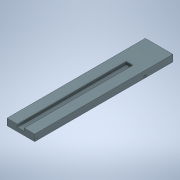
# Autodesk Inventor part: sina
Saved by Autodesk Inventor 2021.2 (Build 252289000, 289)
## iProperties
Created: 2024-04-19
Part Number: sina
Material: Lead
Document SubType Name: Modeling
Designer: cioba
Density: 11.34 g/cm^3
Appearance: Lead
Author: cioba
Autodesk Inventor part; units mm, degrees
ref_plane "YZ Plane" through (0, 0, 0) normal (1, 0, 0) x (0, 1, 0)
ref_plane "XZ Plane" through (0, 0, 0) normal (0, 1, 0) x (-1, 0, 0)
ref_plane "XY Plane" through (0, 0, 0) normal (0, 0, 1) x (1, 0, 0)
sketch "Sketch1" plane through (0, 0, 0) normal (0, 0, 1) x (1, 0, 0)
  line L0 (-7.378, 4.0507) -> (34.622, 4.0507)
  line L1 (34.622, 4.0507) -> (34.622, -5.9493)
  line L2 (34.622, -5.9493) -> (-7.378, -5.9493)
  line L3 (-7.378, -5.9493) -> (-7.378, 4.0507)
  line L4 (8.622, 4.0507) -> (8.622, 0.0507)
  line L5 (18.622, 4.0507) -> (18.622, 0.0507)
  line L6 (18.622, 0.0507) -> (8.622, 0.0507)
  point P0 (0, 0)
  constraints: 14 end point, 4 perpendicular, 2 parallel, 2 point on line, 1 horizontal
extrude "Extrusion1" add sketch "Sketch1" against normal blind 45
extrude "Extrusion2" add sketch "Sketch1" along normal blind 165 contours L0 L4 L6 L5 L1 L2 L3
sketch "Sketch2" plane through (34.622, -5.9493, -45) normal (1, 0, 0) x (0, 0, -1)
  line L0 (0, 0) -> (0, 10) projected
  line L1 (0, 0) -> (-210, 0) projected
  line L2 (-210, 10) -> (0, 10) projected
  circle A0 centre (-42.793, 2.5) radius 1.5
  point P0 (-45, 5.9493)
  constraints: 1 centre point
hole "Hole1" at (34.622, -3.4493, -2.207) direction (-1, 0, 0) diameter 3 depth 5 tip angle 118
sketch "Sketch3" plane through (34.622, -5.9493, -45) normal (1, 0, 0) x (0, 0, -1)
  line L0 (0, 0) -> (-210, 0) projected
  line L1 (-210, 0) -> (-207.5, 0)
  line L2 (-207.5, 0) -> (-207.5, 2.5)
  circle A0 centre (-207.5, 2.5) radius 1.5
  point P0 (-45, 5.9493)
  dimension "d19" = 2.5
  dimension "d20" = 2.5
  dimension "d21" = 3
  constraints: 4 end point, 1 centre point, 1 coincident, 1 perpendicular, 1 point on line
  measures "d19" distance of L0.end L1.end
  measures "d20" distance of L1.end L2.end
  measures "d21" diameter of A0
hole "Hole2" at (34.622, -3.4493, 162.5) direction (-1, 0, 0) diameter 3 depth 5 tip angle 118
sketch "Sketch4" plane through (-7.378, -5.9493, -45) normal (-1, 0, 0) x (0, 0, 1)
  circle A0 centre (207.5, 2.5) radius 1.5 projected
  circle A1 centre (207.5, 2.5) radius 1.5
  circle A2 centre (42.793, 2.5) radius 1.5 projected
  circle A3 centre (42.793, 2.5) radius 1.5
  point P0 (45, 5.9493)
  constraints: 2 centre point, 2 coincident
hole "Hole3" at (-7.378, -3.4493, 162.5) direction (1, 0, 0) diameter 3 depth 5 tip angle 118
hole "Hole4" at (-7.378, -3.4493, -2.207) direction (1, 0, 0) diameter 3 depth 5 tip angle 118
body "Solid1"
